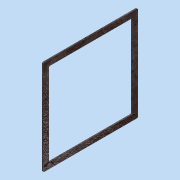
# Autodesk Inventor part: Frontplatte
Saved by Autodesk Inventor 2015 SP1 (Build 190203100, 203)
## iProperties
Created: 2015-04-14
Part Number: Frontplatte
Material: Stahl
Document SubType Name: Modeling
Designer: ElMatinho
Density: 7.85 g/cm^3
Appearance: Unbehandelt
Author: ElMatinho
Autodesk Inventor part; units mm, degrees
ref_plane "YZ Plane" through (0, 0, 0) normal (1, 0, 0) x (0, 1, 0)
ref_plane "XZ Plane" through (0, 0, 0) normal (0, 1, 0) x (-1, 0, 0)
ref_plane "XY Plane" through (0, 0, 0) normal (0, 0, 1) x (1, 0, 0)
sketch "Skizze1" plane through (0, 0, 0) normal (1, 0, 0) x (0, 1, 0)
  line L0 (-176.4, 0) -> (176.4, 0) projected
  line L1 (0, -176.4) -> (0, 176.4) projected
  line L2 (126, 126) -> (-126, 126)
  line L3 (-126, 126) -> (-126, -126)
  line L4 (-126, -126) -> (126, -126)
  line L5 (126, -126) -> (126, 126)
  line L6 (111, 111) -> (-111, 111)
  line L7 (-111, 111) -> (-111, -111)
  line L8 (-111, -111) -> (111, -111)
  line L9 (111, -111) -> (111, 111)
  point P0 (0, 0)
  dimension "d0" = 252
  dimension "d1" = 252
  dimension "d2" = 222
  dimension "d3" = 222
  constraints: 16 end point, 4 parallel, 2 horizontal, 2 perpendicular, 4 other
  measures "d0" distance of L4.end L2.start
  measures "d1" distance of L2.start L2.end
  measures "d2" distance of L8.end L6.start
  measures "d3" distance of L6.start L6.end
extrude "Extrusion1" add sketch "Skizze1" along normal mid plane 3 contours L3 L2 L1 L6 L7 L0 | L0 L7 L8 L1 L4 L3 | L2 L5 L0 L9 L6 L1 | L1 L8 L9 L0 L5 L4
fillet "Rundung1" radius 3 4 edges at (0, 126, 126) (0, 126, -126) (0, -126, -126) (0, -126, 126)
fillet "Rundung2" radius 3 4 edges at (0, -111, -111) (0, 111, -111) (0, 111, 111) (0, -111, 111)
